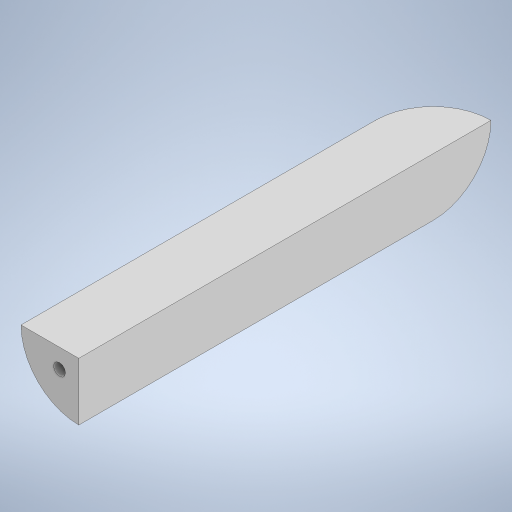
# Autodesk Inventor part: уголок насу
Saved by Autodesk Inventor 2023.1 (Build 271208000, 208)
## iProperties
Created: 2023-02-12
Part Number: уголок насу
Material: Типовые
Document SubType Name: Modeling
Designer: User
Density: 1 g/cm^3
Appearance: По умолчанию
Author: User
Autodesk Inventor part; units mm, degrees
ref_plane "YZ Plane" through (0, 0, 0) normal (1, 0, 0) x (0, 1, 0)
ref_plane "XZ Plane" through (0, 0, 0) normal (0, 1, 0) x (-1, 0, 0)
ref_plane "XY Plane" through (0, 0, 0) normal (0, 0, 1) x (1, 0, 0)
sketch "Эскиз1" plane through (0, 0, 0) normal (0, 0, 1) x (1, 0, 0)
  arc A0 (-15, 0) -> (0, -15) centre (0, 0) ccw
  line L0 (-15, 0) -> (0, 0)
  line L1 (0, 0) -> (0, -15)
  dimension "d0" = 30
  constraints: 4 end point, 2 point on circle, 1 centre point, 1 coincident, 1 horizontal, 1 perpendicular
  measures "d0" diameter of A0
extrude "Выдавливание1" add sketch "Эскиз1" along normal blind 107
fillet "Сопряжение1" radius 15 1 edges at (-10.6066, -10.6066, 0)
sketch "Эскиз2" plane through (0, 0, 107) normal (0, 0, 1) x (1, 0, 0)
  circle A0 centre (-5, -5) radius 1.55
  line L0 (0, 0) -> (-15, 0) projected
  line L1 (0, -15) -> (0, 0) projected
  dimension "d4" = 3.1
  dimension "d5" = 5
  dimension "d6" = 5
  constraints: 1 centre point
  measures "d4" diameter of A0
  measures "d5" distance from line of A0.centre L0
  measures "d6" distance from line of A0.centre L1
extrude "Выдавливание2" cut sketch "Эскиз2" against normal blind 7
